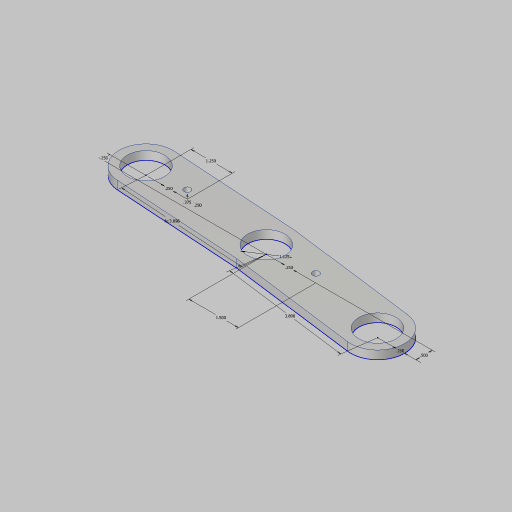
# Autodesk Inventor part: GP3-004
Saved by Autodesk Inventor 2023.5 (Build 275446000, 446)
## iProperties
Created: 2025-02-23
Part Number: GP3-004
Material: Aluminum 6061
Document SubType Name: Modeling
Designer: slick
Density: 2.7 g/cm^3
Appearance: Aluminum - Flat
Author: slick
Autodesk Inventor part; units mm, degrees
ref_plane "YZ Plane" through (0, 0, 0) normal (1, 0, 0) x (0, 1, 0)
ref_plane "XZ Plane" through (0, 0, 0) normal (0, 1, 0) x (-1, 0, 0)
ref_plane "XY Plane" through (0, 0, 0) normal (0, 0, 1) x (1, 0, 0)
sketch "Sketch1" plane through (0, 0, 0) normal (0, 1, 0) x (-1, 0, 0)
  circle A0 centre (0, 0) radius 14.2875
  circle A1 centre (-98.1811, 12.7) radius 14.2875
  circle A2 centre (98.7952, -6.35) radius 14.2875
  circle A3 centre (98.7952, -6.35) radius 20.6375 construction
  circle A4 centre (0, 0) radius 20.6375 construction
  circle A5 centre (-98.1811, 12.7) radius 20.6375 construction
  circle A6 centre (67.0452, -6.35) radius 4.7625 construction
  circle A7 centre (-38.1, 0) radius 4.7625 construction
  circle A8 centre (67.0452, -6.35) radius 11.1125 construction
  circle A9 centre (-38.1, 0) radius 11.1125 construction
  line L0 (100.1189, 14.245) -> (1.3237, 20.595)
  line L1 (2.6475, 20.467) -> (-95.5336, 33.167)
  line L2 (-100.8285, -7.767) -> (-2.6475, -20.467)
  line L3 (97.4714, -26.945) -> (-1.3237, -20.595)
  arc A10 (-2.6475, -20.467) -> (-1.3237, -20.595) centre (0, 0) ccw
  arc A11 (97.4714, -26.945) -> (100.1189, 14.245) centre (98.7952, -6.35) ccw
  arc A12 (-95.5336, 33.167) -> (-100.8285, -7.767) centre (-98.1811, 12.7) ccw
  point P0 (1.9877, 20.5523)
  dimension "d0" = 28.575
  dimension "d1" = 98.999
  dimension "d2" = 98.999
  dimension "d3" = 12.7
  dimension "d4" = 6.35
  dimension "d5" = 6.35
  dimension "d6" = 6.35
  dimension "d7" = 6.35
  dimension "d8" = 31.75
  dimension "d9" = 38.1
  dimension "d10" = 9.525
  dimension "d11" = 6.35
  constraints: 14 point on circle, 13 centre point, 8 end point, 8 tangent, 6 coincident, 4 equal radius, 2 horizontal alignment
  measures "d0" diameter of A0
  measures "d1" distance of A1.centre point (0, 0)
  measures "d2" distance of A2.centre point (0, 0)
  measures "d3" vertical distance of A1.centre point (0, 0)
  measures "d4" vertical distance of A2.centre point (0, 0)
  measures "d5" radial gap between concentric circles of A2 A3
  measures "d6" radial gap between concentric circles of A0 A4
  measures "d7" radial gap between concentric circles of A1 A5
  measures "d8" distance of point (67.045, -6.35) A2.centre
  measures "d9" distance of point (-38.1, 0) point (0, 0)
  measures "d10" diameter of A6
  measures "d11" radial gap between concentric circles of A6 A8
extrude "Extrusion1" add sketch "Sketch1" along normal blind 6.35
hole "Hole1" at (38.1, 0, 0) at (-67.0452, 0, -6.35) direction (0, 1, 0) diameter 5.1054 end through all clearance for "Flat Head Machine Screw (82)" size "#10" standard "Ansi Unified Screw Threads"
equation "\"d2\" = d1"
body "Solid1"
